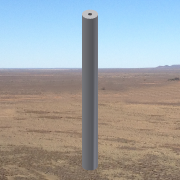
# Autodesk Inventor part: 2f1ds
Saved by Autodesk Inventor 2014 SP1 (Build 180222100, 222)
## iProperties
Company: HERA Project
Created: 2013-06-03
Part Number: 2f1ds
Material: Acetal Resin, White
Document SubType Name: Modeling
Designer: Rich Bradley
Density: 1.425 g/cm^3
Description: Feed disk spacer
Mass: 26.3641 g
Surface Area: 60.8049 cm^2
Volume: 18.5012 cm^3
Appearance: Smooth - White
Author: David DeBoer
Title: Feed spacer
Autodesk Inventor part; units mm, degrees
ref_plane "YZ Plane" through (0, 0, 0) normal (1, 0, 0) x (0, 1, 0)
ref_plane "XZ Plane" through (0, 0, 0) normal (0, 1, 0) x (-1, 0, 0)
ref_plane "XY Plane" through (0, 0, 0) normal (0, 0, 1) x (1, 0, 0)
sketch "Sketch1" plane through (0, 0, 0) normal (0, 1, 0) x (-1, 0, 0)
  circle A0 centre (0, 0) radius 6.35
  dimension "d0" = 12.7
  constraints: 1 centre point, 1 coincident
  measures "d0" diameter of A0
extrude "Extrusion1" add sketch "Sketch1" along normal blind 146.05
sketch "Sketch2" plane through (0, 146.05, 0) normal (0, 1, 0) x (1, 0, 0)
  circle A0 centre (0, 0) radius 6.35 projected
  circle A1 centre (0, 0) radius 1.7528
  constraints: 1 centre point, 1 coincident
hole "Hole1" at (0, 146.05, 0) direction (0, -1, 0) diameter 3.302 depth 15.24 tip angle 118 thread size "8-32 UNC" class "2B" standard "ANSI Unified Screw Threads"
sketch "Sketch3" plane through (0, 0, 0) normal (0, -1, 0) x (1, 0, 0)
  circle A0 centre (0, 0) radius 6.35 projected
  circle A1 centre (0, 0) radius 2.7242
  constraints: 1 centre point, 1 coincident
hole "Hole2" at (0, 0, 0) direction (0, 1, 0) diameter 3.302 depth 15.24 tip angle 118 thread size "8-32 UNC" class "2B" standard "ANSI Unified Screw Threads"
body "Solid1"
